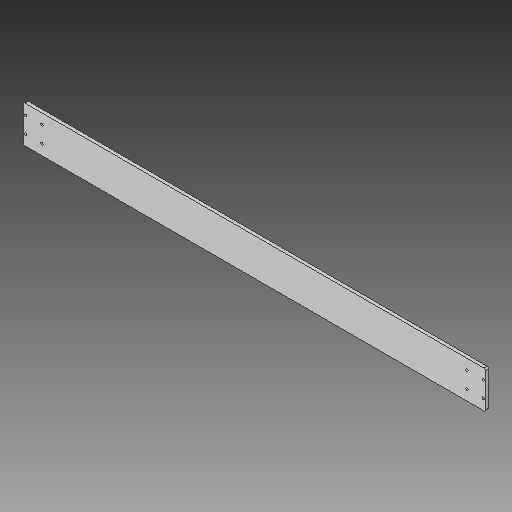
# Autodesk Inventor part: Wiper_Arm_1
Saved by Autodesk Inventor 2019 (Build 230136000, 136)
## iProperties
Created: 2020-03-11
Part Number: Wiper_Arm_1
Material: Generic
Document SubType Name: Modeling
Designer: Vijay
Density: 1 g/cm^3
Appearance: Default
Author: Vijay
Autodesk Inventor part; units mm, degrees
ref_plane "YZ Plane" through (0, 0, 0) normal (1, 0, 0) x (0, 1, 0)
ref_plane "XZ Plane" through (0, 0, 0) normal (0, 1, 0) x (-1, 0, 0)
ref_plane "XY Plane" through (0, 0, 0) normal (0, 0, 1) x (1, 0, 0)
sketch "Sketch1" plane through (0, 0, 0) normal (0, 0, 1) x (1, 0, 0)
  line L0 (19.3, -32.4001) -> (25.8, -32.4001) construction
  line L1 (25.8, -0.0001) -> (25.8, -32.4001) construction
  line L2 (19.3, -0.0001) -> (25.8, -0.0001) construction
  line L3 (19.3, -0.0001) -> (19.3, -32.4001) construction
  circle A0 centre (22.9, -6.2001) radius 1.75 construction
  circle A1 centre (22.9, -26.2001) radius 1.75 construction
  line L4 (0, -32.4001) -> (6.5, -32.4001) construction
  line L5 (6.5, -0.0001) -> (6.5, -32.4001) construction
  line L6 (0, -0.0001) -> (6.5, -0.0001) construction
  line L7 (0, 0) -> (0, -32.4001) projected
  circle A2 centre (2.9, -6.2001) radius 1.75 construction
  circle A3 centre (2.9, -26.2001) radius 1.75 construction
  line L8 (560.3003, -32.4001) -> (566.8003, -32.4001) construction
  line L9 (566.8003, -0.0001) -> (566.8003, -32.4001) projected
  line L10 (560.3003, -0.0001) -> (566.8003, -0.0001) construction
  line L11 (560.3003, -0.0001) -> (560.3003, -32.4001) construction
  circle A4 centre (563.9003, -6.2001) radius 1.75 construction
  circle A5 centre (563.9003, -26.2001) radius 1.75 construction
  line L12 (541.0003, -32.4001) -> (547.5003, -32.4001) construction
  line L13 (547.5003, -0.0001) -> (547.5003, -32.4001) construction
  line L14 (541.0003, -0.0001) -> (547.5003, -0.0001) construction
  line L15 (541.0003, -0.0001) -> (541.0003, -32.4001) construction
  circle A6 centre (543.9003, -6.2001) radius 1.75 construction
  circle A7 centre (543.9003, -26.2001) radius 1.75 construction
  line L16 (541.9003, 6.4999) -> (565.9003, 6.4999) projected
  line L17 (565.9003, -38.9001) -> (541.9003, -38.9001) projected
  line L18 (566.7649, -38.9) -> (0, -38.9)
  line L19 (0, -38.9) -> (0, 6.5)
  line L20 (0, 6.5) -> (566.7649, 6.5)
  line L21 (566.7649, 6.5) -> (566.7649, -38.9)
  circle A8 centre (563.9003, -26.2001) radius 1.5
  circle A9 centre (563.9003, -6.2001) radius 1.5
  circle A10 centre (543.9003, -26.2001) radius 1.5
  circle A11 centre (543.9003, -6.2001) radius 1.5
  circle A12 centre (22.9, -26.2001) radius 1.5
  circle A13 centre (22.9, -6.2001) radius 1.5
  circle A14 centre (2.9, -26.2001) radius 1.5
  circle A15 centre (2.9, -6.2001) radius 1.5
  dimension "d0" = 3
  dimension "d1" = 3
  dimension "d2" = 3
  dimension "d3" = 3
  dimension "d4" = 3
  dimension "d5" = 3
  dimension "d6" = 3
  dimension "d7" = 3
  constraints: 8 centre point, 8 coincident, 8 end point, 2 parallel, 1 horizontal, 1 perpendicular
  measures "d0" diameter of A8
  measures "d1" diameter of A9
  measures "d2" diameter of A10
  measures "d3" diameter of A11
  measures "d4" diameter of A12
  measures "d5" diameter of A13
  measures "d6" diameter of A14
  measures "d7" diameter of A15
extrude "Extrusion1" add sketch "Sketch1" along normal blind 4
fillet "Fillet1" radius 2 4 edges at (566.7649, 6.5, 2) (566.7649, -38.9, 2) (0, -38.9, 2) (0, 6.5, 2)
body "Solid1"
